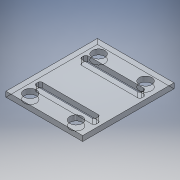
# Autodesk Inventor part: КВ33.000.105 - Заслонка
Saved by Autodesk Inventor 2019 (Build 230136000, 136)
## iProperties
Created: 2021-03-17
Part Number: КВ33.000.105 - Заслонка
Material: Типовые
Document SubType Name: Modeling
Designer: Петров Иван
Density: 1 g/cm^3
Appearance: Clear
Author: Петров Иван
Autodesk Inventor part; units mm, degrees
ref_plane "YZ Plane" through (0, 0, 0) normal (1, 0, 0) x (0, 1, 0)
ref_plane "XZ Plane" through (0, 0, 0) normal (0, 1, 0) x (-1, 0, 0)
ref_plane "XY Plane" through (0, 0, 0) normal (0, 0, 1) x (1, 0, 0)
sketch "Sketch1" plane through (0, 0, 0) normal (0, 1, 0) x (-1, 0, 0)
  line L0 (58.5724, -67.15) -> (66.5724, -67.15) projected
  line L1 (58.5724, 20.85) -> (58.5724, -67.15) projected
  line L2 (66.5724, 20.85) -> (58.5724, 20.85) projected
  line L3 (66.5724, 20.85) -> (66.5724, -67.15) projected
  line L4 (-7.3261, 20.85) -> (0.6739, 20.85) projected
  line L5 (-7.3261, -67.15) -> (-7.3261, 20.85) projected
  line L6 (0.6739, -67.15) -> (-7.3261, -67.15) projected
  line L7 (0.6739, 20.85) -> (0.6739, -67.15) projected
  line L8 (58.5724, 20.85) -> (0.6739, 20.85)
  line L9 (58.5724, -67.15) -> (0.6739, -67.15)
  point P0 (0, 0)
  constraints: 4 end point, 1 collinear, 1 horizontal
extrude "Extrusion1" add sketch "Sketch1" against normal blind 5
sketch "Sketch2" plane through (0, -5, 0) normal (0, -1, 0) x (1, 0, 0)
  line L0 (-58.5724, 20.85) -> (-58.5724, -67.15) projected
  line L1 (-0.6739, -67.15) -> (-0.6739, 20.85) projected
  line L2 (-79.1232, -42.15) -> (-79.1232, -48.15) projected
  line L3 (-79.1232, 1.85) -> (-79.1232, -4.15) projected
  line L4 (-79.1232, 1.85) -> (-0.6739, 1.85)
  line L5 (-0.6739, 1.85) -> (-0.6739, -4.15)
  line L6 (-0.6739, -4.15) -> (-79.1232, -4.15)
  line L7 (-79.1232, -4.15) -> (-79.1232, 1.85)
  line L8 (-79.1232, -42.15) -> (-0.6739, -42.15)
  line L9 (-0.6739, -42.15) -> (-0.6739, -48.15)
  line L10 (-0.6739, -48.15) -> (-79.1232, -48.15)
  line L11 (-79.1232, -48.15) -> (-79.1232, -42.15)
  line L12 (-58.5724, 1.85) -> (-58.5724, -4.15)
  line L13 (-58.5724, -42.15) -> (-58.5724, -48.15)
  point P0 (0, 0)
  point P1 (-0.6739, -2.6877)
  point P2 (-58.5724, -2.6877)
  point P3 (-0.6739, -8.6877)
  point P4 (-58.5724, -8.6877)
  constraints: 20 end point, 14 point on line, 4 parallel, 2 horizontal, 2 perpendicular, 4 other
extrude "Extrusion2" cut sketch "Sketch2" against normal blind 5 contours L4 L1 L6 L0 | L8 L1 L10 L0
fillet "Fillet1" radius 2 8 edges at (-58.5724, -2.5, 1.85) (-58.5724, -2.5, -4.15) (-0.6739, -2.5, 1.85) (-0.6739, -2.5, -4.15) (-0.6739, -2.5, -42.15) (-0.6739, -2.5, -48.15) (-58.5724, -2.5, -42.15) (-58.5724, -2.5, -48.15)
sketch "Sketch3" plane through (0, -5, 0) normal (0, -1, 0) x (1, 0, 0)
  circle A0 centre (-8.8162, 11.0267) radius 6 projected
  circle A1 centre (-53.0208, 11.0267) radius 6 projected
  circle A2 centre (-53.0208, -54.8709) radius 6 projected
  circle A3 centre (-7.7929, -54.8709) radius 6 projected
  point P0 (0, 0)
extrude "Extrusion3" cut sketch "Sketch3" against normal blind 10
body "Solid1"
